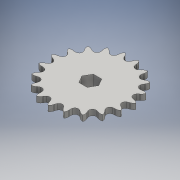
# Autodesk Inventor part: sprocket19teeth
Saved by Autodesk Inventor 2016 (Build 200138000, 138)
## iProperties
Created: 2016-10-16
Part Number: sprocket19teeth
Material: Generic
Document SubType Name: Modeling
Designer: Kevin G
Density: 1 g/cm^3
Appearance: Default
Author: Kevin G
Autodesk Inventor part; units mm, degrees
ref_plane "YZ Plane" through (0, 0, 0) normal (1, 0, 0) x (0, 1, 0)
ref_plane "XZ Plane" through (0, 0, 0) normal (0, 1, 0) x (-1, 0, 0)
ref_plane "XY Plane" through (0, 0, 0) normal (0, 0, 1) x (1, 0, 0)
sketch "Sketch1" plane through (0, 0, 0) normal (0, 0, 1) x (1, 0, 0)
  arc A0 (-2.9258, 28.8351) -> (-2.0289, 27.3418) centre (3.1785, 31.4854) ccw
  arc A1 (-3.1688, 29.4047) -> (-5.2669, 31.5626) centre (-7.0155, 27.7636) ccw
  line L0 (-2.9258, 28.8351) -> (-3.1688, 29.4047)
  line L1 (0, 28.9359) -> (0, 28.9345)
  arc A2 (-2.0289, 27.3418) -> (0, 26.3551) centre (0, 28.9345) ccw
  arc A3 (2.0289, 27.3418) -> (2.9258, 28.8351) centre (-3.1785, 31.4854) ccw
  arc A4 (5.2669, 31.5626) -> (3.1688, 29.4047) centre (7.0155, 27.7636) ccw
  line L2 (2.9258, 28.8351) -> (3.1688, 29.4047)
  arc A5 (0, 26.3551) -> (2.0289, 27.3418) centre (0, 28.9345) ccw
  arc A6 (-12.5448, 26.7826) -> (-15.2298, 28.1423) centre (-15.6502, 23.9813) ccw
  arc A7 (-10.7968, 25.2015) -> (-8.5575, 24.9271) centre (-9.395, 27.3667) ccw
  arc A8 (-12.13, 26.3227) -> (-10.7968, 25.2015) centre (-7.217, 30.8115) ccw
  line L3 (-12.13, 26.3227) -> (-12.5448, 26.7826)
  arc A9 (-8.5575, 24.9271) -> (-6.9589, 26.5191) centre (-9.395, 27.3667) ccw
  arc A10 (-6.9589, 26.5191) -> (-6.5955, 28.2227) centre (-13.2296, 28.7474) ccw
  arc A11 (-5.2669, 31.5626) -> (-6.5506, 28.8404) centre (-2.3795, 28.5372) ccw
  line L4 (-6.5955, 28.2227) -> (-6.5506, 28.8404)
  arc A12 (-20.5614, 21.2581) -> (-23.5424, 21.6723) centre (-22.5889, 17.6004) ccw
  arc A13 (-18.3947, 20.3303) -> (-16.1877, 20.7979) centre (-17.7719, 22.8334) ccw
  arc A14 (-20.0198, 20.9579) -> (-18.3947, 20.3303) centre (-16.8305, 26.7987) ccw
  line L5 (-20.0198, 20.9579) -> (-20.5614, 21.2581)
  arc A15 (-16.1877, 20.7979) -> (-15.1926, 22.8227) centre (-17.7719, 22.8334) ccw
  arc A16 (-15.1926, 22.8227) -> (-15.402, 24.552) centre (-21.847, 22.8942) ccw
  arc A17 (-15.2298, 28.1423) -> (-15.5601, 25.1508) centre (-11.5165, 26.2183) ccw
  line L6 (-15.402, 24.552) -> (-15.5601, 25.1508)
  arc A18 (-26.3498, 13.43) -> (-29.3038, 12.8539) centre (-27.0798, 9.3121) ccw
  arc A19 (-23.9993, 13.256) -> (-22.0636, 14.4149) centre (-24.223, 15.8257) ccw
  arc A20 (-25.74, 13.3219) -> (-23.9993, 13.256) centre (-24.6201, 19.8818) ccw
  line L7 (-25.74, 13.3219) -> (-26.3498, 13.43)
  arc A21 (-22.0636, 14.4149) -> (-21.7799, 16.653) centre (-24.223, 15.8257) ccw
  arc A22 (-21.7799, 16.653) -> (-22.5395, 18.2207) centre (-28.097, 14.56) ccw
  arc A23 (-23.5424, 21.6723) -> (-22.8835, 18.7357) centre (-19.4056, 21.0584) ccw
  line L8 (-22.5395, 18.2207) -> (-22.8835, 18.7357)
  arc A24 (-29.2828, 4.1466) -> (-31.8897, 2.6425) centre (-28.6362, 0.0147) ccw
  arc A25 (-27.0032, 4.7452) -> (-25.5487, 6.4698) centre (-28.0491, 7.103) ccw
  arc A26 (-28.671, 4.2423) -> (-27.0032, 4.7452) centre (-29.7417, 10.8104) ccw
  line L9 (-28.671, 4.2423) -> (-29.2828, 4.1466)
  arc A27 (-25.5487, 6.4698) -> (-26.0071, 8.6788) centre (-28.0491, 7.103) ccw
  arc A28 (-26.0071, 8.6788) -> (-27.2345, 9.9149) centre (-31.3022, 4.648) ccw
  arc A29 (-29.3038, 12.8539) -> (-27.727, 10.2903) centre (-25.1918, 13.6164) ccw
  line L10 (-27.2345, 9.9149) -> (-27.727, 10.2903)
  arc A30 (-29.0426, -5.5862) -> (-31.0198, -7.8553) centre (-27.0894, -9.2842) ccw
  arc A31 (-27.0808, -4.2798) -> (-26.2651, -2.1764) centre (-28.8357, -2.3894) ccw
  arc A32 (-28.495, -5.297) -> (-27.0808, -4.2798) centre (-31.6404, 0.5676) ccw
  line L11 (-28.495, -5.297) -> (-29.0426, -5.5862)
  arc A33 (-26.2651, -2.1764) -> (-27.4159, -0.2359) centre (-28.8357, -2.3894) ccw
  arc A34 (-27.4159, -0.2359) -> (-28.9782, 0.5346) centre (-31.1154, -5.7677) ccw
  arc A35 (-31.8897, 2.6425) -> (-29.5659, 0.7298) centre (-28.2481, 4.6988) ccw
  line L12 (-28.9782, 0.5346) -> (-29.5659, 0.7298)
  arc A36 (-25.6551, -14.7136) -> (-26.7885, -17.5018) centre (-22.607, -17.5771) ccw
  arc A37 (-24.2239, -12.8411) -> (-24.1353, -10.5867) centre (-26.4974, -11.6229) ccw
  arc A38 (-25.2311, -14.2623) -> (-24.2239, -12.8411) centre (-30.1103, -9.7368) ccw
  line L13 (-25.2311, -14.2623) -> (-25.6551, -14.7136)
  arc A39 (-24.1353, -10.5867) -> (-25.8539, -9.1251) centre (-26.4974, -11.6229) ccw
  arc A40 (-25.8539, -9.1251) -> (-27.5817, -8.9036) centre (-27.5567, -15.5583) ccw
  arc A41 (-31.0198, -7.8553) -> (-28.2009, -8.9098) centre (-28.2432, -4.7279) ccw
  line L14 (-27.5817, -8.9036) -> (-28.2009, -8.9098)
  arc A42 (-19.4876, -22.2466) -> (-19.6542, -25.2517) centre (-15.6749, -23.9652) ccw
  arc A43 (-18.7419, -20.0108) -> (-19.3901, -17.8498) centre (-21.2878, -19.5968) ccw
  arc A44 (-19.2331, -21.6821) -> (-18.7419, -20.0108) centre (-25.3173, -18.986) ccw
  line L15 (-19.2331, -21.6821) -> (-19.4876, -22.2466)
  arc A45 (-19.3901, -17.8498) -> (-21.4901, -17.0254) centre (-21.2878, -19.5968) ccw
  arc A46 (-21.4901, -17.0254) -> (-23.1963, -17.3769) centre (-21.0118, -23.663) ccw
  arc A47 (-26.7885, -17.5018) -> (-23.7799, -17.5839) centre (-25.1778, -13.6423) ccw
  line L16 (-23.1963, -17.3769) -> (-23.7799, -17.5839)
  arc A48 (-11.2082, -27.3688) -> (-10.3901, -30.2652) centre (-7.0441, -27.7563) ccw
  arc A49 (-11.2289, -25.012) -> (-12.5437, -23.1786) centre (-13.7713, -25.4471) ccw
  arc A50 (-11.1508, -26.7522) -> (-11.2289, -25.012) centre (-17.7808, -26.1778) ccw
  line L17 (-11.1508, -26.7522) -> (-11.2082, -27.3688)
  arc A51 (-12.5437, -23.1786) -> (-14.7976, -23.0807) centre (-13.7713, -25.4471) ccw
  arc A52 (-14.7976, -23.0807) -> (-16.2972, -23.9672) centre (-12.19, -29.2034) ccw
  arc A53 (-19.6542, -25.2517) -> (-16.782, -24.3525) centre (-19.3839, -21.0783) ccw
  line L18 (-16.2972, -23.9672) -> (-16.782, -24.3525)
  arc A54 (-1.7143, -29.5252) -> (0, -31.999) centre (2.3501, -28.5396) ccw
  arc A55 (-2.4991, -27.3028) -> (-4.3379, -25.9957) centre (-4.7625, -28.5399) ccw
  arc A56 (-1.8602, -28.9234) -> (-2.4991, -27.3028) centre (-8.3175, -30.5328) ccw
  line L19 (-1.8602, -28.9234) -> (-1.7143, -29.5252)
  arc A57 (-4.3379, -25.9957) -> (-6.5015, -26.6349) centre (-4.7625, -28.5399) ccw
  arc A58 (-6.5015, -26.6349) -> (-7.632, -27.9603) centre (-2.0472, -31.5792) ccw
  arc A59 (-10.3901, -30.2652) -> (-7.9654, -28.4821) centre (-11.4895, -26.2302) ccw
  line L20 (-7.632, -27.9603) -> (-7.9654, -28.4821)
  arc A60 (7.9654, -28.4821) -> (10.3901, -30.2652) centre (11.4895, -26.2302) ccw
  arc A61 (6.5015, -26.6349) -> (4.3379, -25.9957) centre (4.7625, -28.5399) ccw
  arc A62 (7.632, -27.9603) -> (6.5015, -26.6349) centre (2.0472, -31.5792) ccw
  line L21 (7.632, -27.9603) -> (7.9654, -28.4821)
  arc A63 (4.3379, -25.9957) -> (2.4991, -27.3028) centre (4.7625, -28.5399) ccw
  arc A64 (2.4991, -27.3028) -> (1.8602, -28.9234) centre (8.3175, -30.5328) ccw
  arc A65 (0, -31.999) -> (1.7143, -29.5252) centre (-2.3501, -28.5396) ccw
  line L22 (1.8602, -28.9234) -> (1.7143, -29.5252)
  arc A66 (16.782, -24.3525) -> (19.6542, -25.2517) centre (19.3839, -21.0783) ccw
  arc A67 (14.7976, -23.0807) -> (12.5437, -23.1786) centre (13.7713, -25.4471) ccw
  arc A68 (16.2972, -23.9672) -> (14.7976, -23.0807) centre (12.19, -29.2034) ccw
  line L23 (16.2972, -23.9672) -> (16.782, -24.3525)
  arc A69 (12.5437, -23.1786) -> (11.2289, -25.012) centre (13.7713, -25.4471) ccw
  arc A70 (11.2289, -25.012) -> (11.1508, -26.7522) centre (17.7808, -26.1778) ccw
  arc A71 (10.3901, -30.2652) -> (11.2082, -27.3688) centre (7.0441, -27.7563) ccw
  line L24 (11.1508, -26.7522) -> (11.2082, -27.3688)
  arc A72 (23.7799, -17.5839) -> (26.7885, -17.5018) centre (25.1778, -13.6423) ccw
  arc A73 (21.4901, -17.0254) -> (19.3901, -17.8498) centre (21.2878, -19.5968) ccw
  arc A74 (23.1963, -17.3769) -> (21.4901, -17.0254) centre (21.0118, -23.663) ccw
  line L25 (23.1963, -17.3769) -> (23.7799, -17.5839)
  arc A75 (19.3901, -17.8498) -> (18.7419, -20.0108) centre (21.2878, -19.5968) ccw
  arc A76 (18.7419, -20.0108) -> (19.2331, -21.6821) centre (25.3173, -18.986) ccw
  arc A77 (19.6542, -25.2517) -> (19.4876, -22.2466) centre (15.6749, -23.9652) ccw
  line L26 (19.2331, -21.6821) -> (19.4876, -22.2466)
  arc A78 (28.2009, -8.9098) -> (31.0198, -7.8553) centre (28.2432, -4.7279) ccw
  arc A79 (25.8539, -9.1251) -> (24.1353, -10.5867) centre (26.4974, -11.6229) ccw
  arc A80 (27.5817, -8.9036) -> (25.8539, -9.1251) centre (27.5567, -15.5583) ccw
  line L27 (27.5817, -8.9036) -> (28.2009, -8.9098)
  arc A81 (24.1353, -10.5867) -> (24.2239, -12.8411) centre (26.4974, -11.6229) ccw
  arc A82 (24.2239, -12.8411) -> (25.2311, -14.2623) centre (30.1103, -9.7368) ccw
  arc A83 (26.7885, -17.5018) -> (25.6551, -14.7136) centre (22.607, -17.5771) ccw
  line L28 (25.2311, -14.2623) -> (25.6551, -14.7136)
  arc A84 (29.5659, 0.7298) -> (31.8897, 2.6425) centre (28.2481, 4.6988) ccw
  arc A85 (27.4159, -0.2359) -> (26.2651, -2.1764) centre (28.8357, -2.3894) ccw
  arc A86 (28.9782, 0.5346) -> (27.4159, -0.2359) centre (31.1154, -5.7677) ccw
  line L29 (28.9782, 0.5346) -> (29.5659, 0.7298)
  arc A87 (26.2651, -2.1764) -> (27.0808, -4.2798) centre (28.8357, -2.3894) ccw
  arc A88 (27.0808, -4.2798) -> (28.495, -5.297) centre (31.6404, 0.5676) ccw
  arc A89 (31.0198, -7.8553) -> (29.0426, -5.5862) centre (27.0894, -9.2842) ccw
  line L30 (28.495, -5.297) -> (29.0426, -5.5862)
  arc A90 (27.727, 10.2903) -> (29.3038, 12.8539) centre (25.1918, 13.6164) ccw
  arc A91 (26.0071, 8.6788) -> (25.5487, 6.4698) centre (28.0491, 7.103) ccw
  arc A92 (27.2345, 9.9149) -> (26.0071, 8.6788) centre (31.3022, 4.648) ccw
  line L31 (27.2345, 9.9149) -> (27.727, 10.2903)
  arc A93 (25.5487, 6.4698) -> (27.0032, 4.7452) centre (28.0491, 7.103) ccw
  arc A94 (27.0032, 4.7452) -> (28.671, 4.2423) centre (29.7417, 10.8104) ccw
  arc A95 (31.8897, 2.6425) -> (29.2828, 4.1466) centre (28.6362, 0.0147) ccw
  line L32 (28.671, 4.2423) -> (29.2828, 4.1466)
  arc A96 (22.8835, 18.7357) -> (23.5424, 21.6723) centre (19.4056, 21.0584) ccw
  arc A97 (21.7799, 16.653) -> (22.0636, 14.4149) centre (24.223, 15.8257) ccw
  arc A98 (22.5395, 18.2207) -> (21.7799, 16.653) centre (28.097, 14.56) ccw
  line L33 (22.5395, 18.2207) -> (22.8835, 18.7357)
  arc A99 (22.0636, 14.4149) -> (23.9993, 13.256) centre (24.223, 15.8257) ccw
  arc A100 (23.9993, 13.256) -> (25.74, 13.3219) centre (24.6201, 19.8818) ccw
  arc A101 (29.3038, 12.8539) -> (26.3498, 13.43) centre (27.0798, 9.3121) ccw
  line L34 (25.74, 13.3219) -> (26.3498, 13.43)
  arc A102 (15.5601, 25.1508) -> (15.2298, 28.1423) centre (11.5165, 26.2183) ccw
  arc A103 (15.1926, 22.8227) -> (16.1877, 20.7979) centre (17.7719, 22.8334) ccw
  arc A104 (15.402, 24.552) -> (15.1926, 22.8227) centre (21.847, 22.8942) ccw
  line L35 (15.402, 24.552) -> (15.5601, 25.1508)
  arc A105 (16.1877, 20.7979) -> (18.3947, 20.3303) centre (17.7719, 22.8334) ccw
  arc A106 (18.3947, 20.3303) -> (20.0198, 20.9579) centre (16.8305, 26.7987) ccw
  arc A107 (23.5424, 21.6723) -> (20.5614, 21.2581) centre (22.5889, 17.6004) ccw
  line L36 (20.0198, 20.9579) -> (20.5614, 21.2581)
  arc A108 (6.5506, 28.8404) -> (5.2669, 31.5626) centre (2.3795, 28.5372) ccw
  arc A109 (6.9589, 26.5191) -> (8.5575, 24.9271) centre (9.395, 27.3667) ccw
  arc A110 (6.5955, 28.2227) -> (6.9589, 26.5191) centre (13.2296, 28.7474) ccw
  line L37 (6.5955, 28.2227) -> (6.5506, 28.8404)
  arc A111 (8.5575, 24.9271) -> (10.7968, 25.2015) centre (9.395, 27.3667) ccw
  arc A112 (10.7968, 25.2015) -> (12.13, 26.3227) centre (7.217, 30.8115) ccw
  arc A113 (15.2298, 28.1423) -> (12.5448, 26.7826) centre (15.6502, 23.9813) ccw
  line L38 (12.13, 26.3227) -> (12.5448, 26.7826)
  point P0 (0, 0)
  constraints: 228 point on circle, 114 centre point, 78 end point, 1 tangent
extrude "Extrusion1" add sketch "Sketch1" along normal blind 4.2767
sketch "Sketch2" plane through (0, 0, 0) normal (0, 0, -1) x (-1, 0, 0)
  circle A0 centre (0, 0) radius 14
  dimension "d24" = 28
  constraints: 1 centre point, 1 coincident
  measures "d24" diameter of A0
extrude "Extrusion2" add sketch "Sketch2" along normal blind 7.62
sketch "Sketch3" plane through (0, 0, -7.62) normal (0, 0, -1) x (-1, 0, 0)
  line L0 (-6.35, 0) -> (-3.175, 5.4993)
  line L1 (-3.175, 5.4993) -> (3.175, 5.4993)
  line L2 (3.175, 5.4993) -> (6.35, 0)
  line L3 (6.35, 0) -> (3.175, -5.4993)
  line L4 (3.175, -5.4993) -> (-3.175, -5.4993)
  line L5 (-3.175, -5.4993) -> (-6.35, 0)
  point P0 (0, 0)
  point P1 (0, 0)
  constraints: 12 end point, 13 other
emboss "Emboss1" sketch "Sketch3" operation cut depth 15 direction (0, 0, 1)
body "Solid1"
